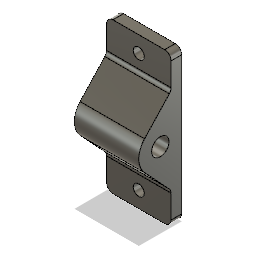
M8_spool_axis v2 (Autodesk Fusion 360 design; units mm, degrees)
Autodesk Fusion 360 part; units mm, degrees
sketch "Sketch1" plane through (0, 0, 0) normal (0, 0, 1) x (1, 0, 0)
  line L0 (15, -35) -> (-15, -35)
  line L1 (-15, -35) -> (-15, 35)
  line L2 (-15, 35) -> (15, 35)
  line L3 (15, 35) -> (15, -35)
  line L4 (15, -35) -> (-15, 35) construction
  line L5 (-15, -35) -> (15, 35) construction
  line L6 (-15, 20) -> (15, 20)
  line L7 (15, 20) -> (15, -20)
  line L8 (15, -20) -> (-15, -20)
  line L9 (-15, -20) -> (-15, 20)
  line L10 (-15, 20) -> (15, -20) construction
  line L11 (15, 20) -> (-15, -20) construction
  line L12 (0, 35) -> (0, 20) construction
  line L13 (0, -20) -> (0, -35) construction
  circle A0 centre (0, -27.5) radius 2.55
  circle A1 centre (0, 27.5) radius 2.55
  dimension "d1" = 30
  dimension "d2" = 15
  dimension "d3" = 40
  dimension "d4" = 5.1
  dimension "d5" = 5.1
  constraint perpendicular L0 L1
  constraint parallel L0 L2
  constraint parallel L1 L3
  constraint horizontal L0
  constraint coincident L4 origin
  constraint coincident L5 origin
  constraint perpendicular L6 L7
  constraint parallel L6 L8
  constraint parallel L7 L9
  constraint horizontal L6
  constraint coincident L1 L6.start
  constraint coincident L10 origin
  constraint coincident L11 origin
  constraint midpoint L2 L12.start
  constraint midpoint L6 L12.end
  constraint midpoint L8 L13.start
  constraint midpoint L0 L13.end
  constraint midpoint L13 A0.centre
  constraint midpoint L12 A1.centre
  measures "d1" distance of L0.start L0.end
  measures "d2" distance of L2 L6
  measures "d3" distance of L6 L8
  measures "d4" diameter of A0
  measures "d5" diameter of A1
extrude "Extrude1" add sketch "Sketch1" along normal blind 5
extrude "Extrude2" add sketch "Sketch1" along normal blind 15 from surface at 5 contours L1 L3 L6 L7 L8 L9
sketch "Sketch2" plane through (15, 0, 0) normal (1, 0, 0) x (0, 0, -1)
  line L0 (0, -35) -> (0, 35)
  line L1 (0, 35) -> (-5, 35)
  line L2 (-5, 35) -> (-5, 20)
  line L3 (-5, 20) -> (-20, 20)
  line L4 (-20, 20) -> (-20, -20)
  line L5 (-20, -20) -> (-5, -20)
  line L6 (-5, -20) -> (-5, -35)
  line L7 (-5, -35) -> (0, -35)
  line L8 (0, 0) -> (-20, 0) construction
  circle A0 centre (-10, 0) radius 4.05
  circle A1 centre (-10, 0) radius 10
  line L9 (-5, 20) -> (-17.3072, 6.8268)
  line L10 (-5, -20) -> (-17.3072, -6.8268)
  dimension "d11" = 8.1
  constraint coincident L8.start origin
  constraint midpoint L4 L8.end
  constraint midpoint L8 A0.centre
  constraint concentric A0 A1
  constraint tangent L4 A1
  constraint coincident L2.end L3.start
  constraint coincident A1 L9.end
  constraint tangent A1 L9
  constraint coincident L5.end L6.start
  constraint coincident A1 L10.end
  constraint tangent A1 L10
  measures "d11" diameter of A0
extrude "Extrude3" cut sketch "Sketch2" against normal through all contours A0
extrude "Extrude8" cut sketch "Sketch2" against normal through all contours L3 L4 A1 L9 | L4 L5 A1 L10
fillet "Fillet1" radius 3 4 edges at (-15, 35, 2.5) (15, 35, 2.5) (-15, -35, 2.5) (15, -35, 2.5)
fillet "Fillet1" radius 3 2 edges at (0, 20, 5) (0, -20, 5)
equation "d4 = d5"
